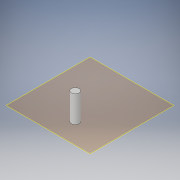
# Autodesk Inventor part: pin_circular_2mm
Saved by Autodesk Inventor 2019 (Build 230136000, 136)
## iProperties
Created: 2018-12-20
Part Number: pin_circular_2mm
Material: Generic
Document SubType Name: Modeling
Designer: assman
Density: 1 g/cm^3
Appearance: Default
Author: assman
Autodesk Inventor part; units mm, degrees
ref_plane "YZ Plane" through (0, 0, 0) normal (1, 0, 0) x (0, 1, 0)
ref_plane "XZ Plane" through (0, 0, 0) normal (0, 1, 0) x (-1, 0, 0)
ref_plane "XY Plane" through (0, 0, 0) normal (0, 0, 1) x (1, 0, 0)
ref_plane "Work Plane1" through (-10, 7, -20) normal (0, 1, 0) x (1, 0, 0)
sketch "Sketch3" plane through (-10, 7, -20) normal (0, 1, 0) x (1, 0, 0)
  circle A0 centre (1.7333, -5.6) radius 1 projected
  point P0 (10, -20)
extrude "Extrusion1" add sketch "Sketch3" along normal blind 7
body "Solid2"
body "Solid1"
